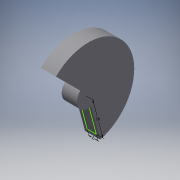
# Autodesk Inventor part: protector
Saved by Autodesk Inventor 2018 (Build 220112000, 112)
## iProperties
Created: 2021-07-10
Part Number: protector
Material: Genérico
Document SubType Name: Modeling
Designer: GABRIEL
Density: 1 g/cm^3
Appearance: Valor por defecto
Author: GABRIEL
Autodesk Inventor part; units mm, degrees
ref_plane "YZ Plane" through (0, 0, 0) normal (1, 0, 0) x (0, 1, 0)
ref_plane "XZ Plane" through (0, 0, 0) normal (0, 1, 0) x (-1, 0, 0)
ref_plane "XY Plane" through (0, 0, 0) normal (0, 0, 1) x (1, 0, 0)
sketch "Boceto1" plane through (0, 0, 0) normal (1, 0, 0) x (0, 1, 0)
  circle A0 centre (0, 0) radius 55
  line L0 (0, 0) -> (-38.8909, 38.8909)
  line L1 (0, 0) -> (55, 0) construction
  line L2 (0, 0) -> (14.235, -53.1259)
  line L3 (0, 0) -> (55, 0) construction
  circle A1 centre (0, 0) radius 20
  dimension "d5" = 110
  dimension "d6" = 135
  dimension "d7" = 75
  dimension "d8" = 40
  constraints: 8 end point, 2 centre point, 2 coincident, 2 equal length, 2 horizontal, 2 point on circle
  measures "d5" diameter of A0
  measures "d6" angle of L1 L0
  measures "d7" angle of L2 L3
  measures "d8" diameter of A1
extrude "Extrusión1" add sketch "Boceto1" along normal blind 10 contours A0 L2 A1 L0 | A1 L2 L0 | L0 L2 A1 picked at (43.0137, -3.4084)
sketch "Boceto2" plane through (0, 5.1764, -19.3185) normal (0, -0.9659258, -0.258819) x (1, 0, 0)
  line L0 (2, -5) -> (8, -5)
  line L1 (8, -5) -> (8, -33)
  line L2 (8, -33) -> (2, -33)
  line L3 (2, -33) -> (2, -5)
  line L4 (10, 0) -> (10, 37.3205) projected
  line L5 (0, -35) -> (10, -35) projected
  point P0 (0, 20)
  dimension "d11" = 6
  dimension "d12" = 28
  dimension "d18" = 2
  constraints: 8 end point, 2 parallel, 1 horizontal, 1 perpendicular
  measures "d11" distance of L1.end L2.end
  measures "d12" distance of L0.end L1.end
  measures "d18" distance between parallel lines of L5 L2
revolve "Revolución1" cut sketch "Boceto2" angle 360 about axis through (2, 6.4705, -24.1481) along (1, 0, 0)
sketch "Boceto3" plane through (10, 0, 0) normal (1, 0, 0) x (0, 0, -1)
  circle A0 centre (0, 0) radius 10
  arc A1 (-14.1421, -14.1421) -> (19.3185, 5.1764) centre (0, 0) ccw projected
  dimension "d20" = 20
  constraints: 1 centre point, 1 concentric
  measures "d20" diameter of A0
extrude "Extrusión2" cut sketch "Boceto3" against normal blind 10
